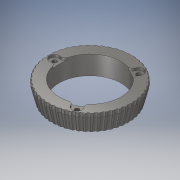
# Autodesk Inventor part: Flywheel Mass
Saved by Autodesk Inventor 2019.4 (Build 234330000, 330)
## iProperties
Created: 2020-02-21
Part Number: Flywheel Mass
Material: Steel, Mild
Document SubType Name: Modeling
Designer: admin
Density: 7.85 g/cm^3
Appearance: Semi-Polished
Author: admin
Autodesk Inventor part; units mm, degrees
ref_plane "YZ Plane" through (0, 0, 0) normal (1, 0, 0) x (0, 1, 0)
ref_plane "XZ Plane" through (0, 0, 0) normal (0, 1, 0) x (-1, 0, 0)
ref_plane "XY Plane" through (0, 0, 0) normal (0, 0, 1) x (1, 0, 0)
sketch "Sketch1" plane through (0, 0, 0) normal (1, 0, 0) x (0, 1, 0)
  line L0 (0, 41.03) -> (25, 41.03)
  line L1 (25, 41.03) -> (25, 55.88)
  line L2 (25, 55.88) -> (20, 55.88)
  line L3 (20, 55.88) -> (0, 50.88)
  line L4 (0, 50.88) -> (0, 41.03)
  line L5 (0, 0) -> (26.8378, 0) construction
  dimension "d0" = 55.88
  dimension "d1" = 5
  dimension "d2" = 25
  dimension "d3" = 20
  dimension "d4" = 41.03
  constraints: 12 end point, 2 horizontal, 2 perpendicular, 1 parallel, 1 point on line
  measures "d0" distance from line of L5.start L2
  measures "d1" vertical distance of L2.end L3.end
  measures "d2" distance of L0.start L0.end
  measures "d3" horizontal distance of L2.end L3.end
  measures "d4" distance from line of L5.start L0
revolve "Revolution1" add sketch "Sketch1" angle 360 about axis through (0, 0, 0) along (0, 1, 0)
sketch "Sketch4" plane through (0, 0, 0) normal (1, 0, 0) x (0, 1, 0)
  line L0 (20, -55.88) -> (25, -55.88) projected
  line L1 (0, -50.88) -> (20, -55.88) projected
  point P0 (0, 0)
sketch "Sketch5" plane through (0, 0, 0) normal (0, -1, 0) x (1, 0, 0)
  circle A0 centre (0, -52) radius 2.5
  line L0 (0, -52) -> (0, 0) construction
  dimension "d25" = 5
  dimension "d26" = 52
  constraints: 2 end point, 1 centre point, 1 vertical
  measures "d25" diameter of A0
  measures "d26" distance of L0.start L0.end
sweep "Sweep1" cut profiles "Sketch5" path "Sketch4" path curves L1
sketch "Sketch6" plane through (0, 25, 0) normal (0, 1, 0) x (1, 0, 0)
  arc A0 (2.2126, 55.8362) -> (-2.2126, 55.8362) centre (0, 0) ccw projected
  arc A1 (-2.2126, 55.8362) -> (2.2126, 55.8362) centre (0, 57) ccw projected
extrude "Extrusion2" cut sketch "Sketch6" against normal through all
pattern_circular "Circular Pattern2" count 50 over 360 about axis through (0, 12.5, 0) along (0, 1, 0) of "Sweep1", "Extrusion2"
sketch "Sketch2" plane through (0, 25, 0) normal (0, 1, 0) x (1, 0, 0)
  circle A0 centre (-47.18, 0) radius 6.65
  circle A1 centre (-47.18, 0) radius 2.75
  line L0 (-47.18, 0) -> (0, 0) construction
  dimension "d6" = 13.3
  dimension "d7" = 5.5
  dimension "d8" = 47.18
  constraints: 2 centre point, 2 end point, 1 coincident, 1 horizontal
  measures "d6" diameter of A0
  measures "d7" diameter of A1
  measures "d8" distance of L0.start L0.end
extrude "Extrusion1" cut sketch "Sketch2" against normal blind 3.1 contours A0 | A1
fillet "Fillet1" radius 5 2 edges at (-40.9622, 23.45, -2.3582) (-40.9622, 23.45, 2.3582)
sketch "Sketch3" plane through (0, 21.9, 0) normal (0, 1, 0) x (1, 0, 0)
  arc A0 (-45.7105, 6.4856) -> (-45.7105, -6.4856) centre (-47.18, 0) ccw projected
  point P0 (0, 0)
  constraints: 1 coincident
hole "Hole1" at (-47.18, 21.9, 0) direction (0, -1, 0) diameter 5.5 end through all
chamfer "Chamfer1" distance 0.5 angle 45 100 edges at (3.1948, 0, -50.7796) (-3.1948, 0, -50.7796) (9.534, 0, -49.9788) (-9.534, 0, -49.9788) (15.7228, 0, -48.3898) (-15.7228, 0, -48.3898) (21.6637, 0, -46.0376) (-21.6637, 0, -46.0376) (27.2629, 0, -42.9594) (-27.2629, 0, -42.9594) (32.4321, 0, -39.2037) (-32.4321, 0, -39.2037) (37.0899, 0, -34.8298) (-37.0899, 0, -34.8298) (41.1628, 0, -29.9065) (-41.1628, 0, -29.9065) (44.5865, 0, -24.5116) (-44.5865, 0, -24.5116) (47.307, 0, -18.7302) (-47.307, 0, -18.7302) (49.2815, 0, -12.6533) (-49.2815, 0, -12.6533) (50.4788, 0, -6.377) (-50.4788, 0, -6.377) (50.88, 0, 0) (-50.88, 0, 0) (50.4788, 0, 6.377) (-50.4788, 0, 6.377) (49.2815, 0, 12.6533) (-49.2815, 0, 12.6533) (47.307, 0, 18.7302) (-47.307, 0, 18.7302) (44.5865, 0, 24.5116) (-44.5865, 0, 24.5116) (41.1628, 0, 29.9065) (-41.1628, 0, 29.9065) (37.0899, 0, 34.8298) (-37.0899, 0, 34.8298) (32.4321, 0, 39.2037) (-32.4321, 0, 39.2037) (27.2629, 0, 42.9594) (-27.2629, 0, 42.9594) (21.6637, 0, 46.0376) (-21.6637, 0, 46.0376) (15.7228, 0, 48.3898) (-15.7228, 0, 48.3898) (9.534, 0, 49.9788) (-9.534, 0, 49.9788) (3.1948, 0, 50.7796) (-3.1948, 0, 50.7796) (-3.5087, 25, 55.7697) (-10.4709, 25, 54.8902) (3.5087, 25, 55.7697) (-17.2679, 25, 53.145) (10.4709, 25, 54.8902) (-23.7925, 25, 50.5617) (17.2679, 25, 53.145) (-29.942, 25, 47.181) (23.7925, 25, 50.5617) (-35.6193, 25, 43.0563) (29.942, 25, 47.181) (-40.7348, 25, 38.2525) (35.6193, 25, 43.0563) (-45.2079, 25, 32.8454) (40.7348, 25, 38.2525) (-48.968, 25, 26.9204) (45.2079, 25, 32.8454) (-51.9559, 25, 20.5708) (48.968, 25, 26.9204) (-54.1244, 25, 13.8968) (51.9559, 25, 20.5708) (-55.4394, 25, 7.0036) (54.1244, 25, 13.8968) (-55.88, 25, 0) (55.4394, 25, 7.0036) (-55.4394, 25, -7.0036) (55.88, 25, 0) (-54.1244, 25, -13.8968) (55.4394, 25, -7.0036) (-51.9559, 25, -20.5708) (54.1244, 25, -13.8968) (-48.968, 25, -26.9204) (51.9559, 25, -20.5708) (-45.2079, 25, -32.8454) (48.968, 25, -26.9204) (-40.7348, 25, -38.2525) (45.2079, 25, -32.8454) (-35.6193, 25, -43.0563) (40.7348, 25, -38.2525) (-29.942, 25, -47.181) (35.6193, 25, -43.0563) (-23.7925, 25, -50.5617) (29.942, 25, -47.181) (-17.2679, 25, -53.145) (23.7925, 25, -50.5617) (-10.4709, 25, -54.8902) (17.2679, 25, -53.145) (-3.5087, 25, -55.7697) (10.4709, 25, -54.8902) (3.5087, 25, -55.7697)
pattern_circular "Circular Pattern1" count 3 over 360 about axis through (0, 12.5, 0) along (0, 1, 0) of "Extrusion1", "Hole1", "Fillet1"
body "Solid1"
